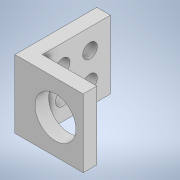
# Autodesk Inventor part: sideSupport
Saved by Autodesk Inventor 2022.2 (Build 262287010, 287A)
## iProperties
Created: 2022-09-12
Part Number: sideSupport
Material: Generic
Document SubType Name: Modeling
Designer: robst
Density: 1 g/cm^3
Appearance: Default
Author: robst
Autodesk Inventor part; units mm, degrees
ref_plane "YZ Plane" through (0, 0, 0) normal (1, 0, 0) x (0, 1, 0)
ref_plane "XZ Plane" through (0, 0, 0) normal (0, 1, 0) x (-1, 0, 0)
ref_plane "XY Plane" through (0, 0, 0) normal (0, 0, 1) x (1, 0, 0)
sketch "Sketch1" plane through (0, 0, 0) normal (1, 0, 0) x (0, 1, 0)
  line L0 (-15.875, 19.05) -> (-15.875, -19.05)
  line L1 (-15.875, -19.05) -> (15.875, -19.05)
  line L2 (15.875, -19.05) -> (15.875, 19.05)
  line L3 (15.875, 19.05) -> (-15.875, 19.05)
  line L4 (-15.875, 19.05) -> (15.875, -19.05) construction
  line L5 (-15.875, -19.05) -> (15.875, 19.05) construction
  point P0 (0, 0)
  dimension "d0" = 31.75
  dimension "d1" = 38.1
  constraints: 12 end point, 2 midpoint, 2 parallel, 1 perpendicular, 1 vertical
  measures "d0" distance of L0.end L1.end
  measures "d1" distance of L1.end L2.end
extrude "Extrusion1" add sketch "Sketch1" against normal blind 6.35
sketch "Sketch2" plane through (0, 0, 0) normal (1, 0, 0) x (0, 0, -1)
  line L0 (-19.05, -15.875) -> (-19.05, 15.875) projected
  line L1 (19.05, -15.875) -> (-19.05, -15.875) projected
  line L2 (-19.05, 15.875) -> (-12.7, 15.875)
  line L3 (-12.7, 15.875) -> (-12.7, -15.875)
  line L4 (-12.7, -15.875) -> (-19.05, -15.875)
  line L5 (-19.05, -15.875) -> (-19.05, 15.875)
  point P0 (0, 0)
  dimension "d4" = 6.35
  constraints: 8 end point, 2 parallel, 1 horizontal, 1 perpendicular, 1 point on line
  measures "d4" distance of L0.end L2.end
extrude "Extrusion2" add sketch "Sketch2" along normal blind 25.4
sketch "Sketch3" plane through (-6.35, -15.875, 19.05) normal (0, 0, 1) x (1, 0, 0)
  circle A0 centre (18.8501, 15.875) radius 9.525
  line L0 (0, 0) -> (0, 31.75) projected
  line L1 (31.75, 31.75) -> (31.75, 0) construction
  line L2 (31.75, 15.875) -> (0, 15.875) construction
  line L3 (0, 31.75) -> (0, 0) construction
  point P0 (6.35, 15.875)
  dimension "d7" = 18.8501
  dimension "d8" = 19.05
  dimension "d11" = 0
  constraints: 2 end point, 2 midpoint, 1 centre point
  measures "d7" distance from line of A0.centre L0
  measures "d8" diameter of A0
  measures "d11" distance from line of A0.centre L2
extrude "Extrusion3" cut sketch "Sketch3" against normal through all
sketch "Sketch4" plane through (0, 0, 0) normal (1, 0, 0) x (0, 0, -1)
  line L0 (9.525, 6.35) -> (-3.175, 6.35) construction
  line L1 (-3.175, 6.35) -> (-3.175, -6.35) construction
  line L2 (-3.175, -6.35) -> (9.525, -6.35) construction
  line L3 (9.525, -6.35) -> (9.525, 6.35) construction
  line L4 (19.05, 15.875) -> (-12.7, 15.875) projected
  line L5 (19.05, -15.875) -> (19.05, 15.875) projected
  line L6 (-12.7, -15.875) -> (-12.7, 15.875) projected
  line L7 (-12.7, -15.875) -> (19.05, -15.875) projected
  point P0 (0, 0)
  dimension "d12" = 9.525
  dimension "d13" = 9.525
  dimension "d14" = 9.525
  dimension "d15" = 9.525
  constraints: 8 end point, 4 coincident, 2 parallel, 1 horizontal, 1 perpendicular
  measures "d12" distance between parallel lines of L0 L4
  measures "d13" distance between parallel lines of L3 L5
  measures "d14" distance between parallel lines of L1 L6
  measures "d15" distance between parallel lines of L2 L7
hole "Hole1" at (0, 6.35, 3.175) at (0, 6.35, -9.525) at (0, -6.35, -9.525) at (0, -6.35, 3.175) direction (-1, 0, 0) diameter 6.7564 end through all clearance for "Hex Machine Screw" size "1/4" standard "Ansi Unified Screw Threads"
body "Solid1"
